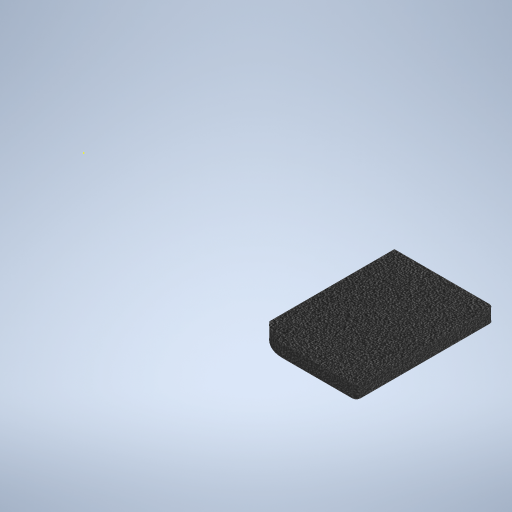
# Autodesk Inventor part: Calco
Saved by Autodesk Inventor 2024 (Build 280153000, 153)
## iProperties
Created: 2024-10-14
Part Number: Calco
Material: Genérico
Document SubType Name: Modeling
Designer: robof
Density: 1 g/cm^3
Appearance: Padrão
Author: robof
Autodesk Inventor part; units mm, degrees
ref_plane "YZ Plane" through (0, 0, 0) normal (1, 0, 0) x (0, 1, 0)
ref_plane "XZ Plane" through (0, 0, 0) normal (0, 1, 0) x (-1, 0, 0)
ref_plane "XY Plane" through (0, 0, 0) normal (0, 0, 1) x (1, 0, 0)
sketch "Esboço1" plane through (0, 0, 0) normal (0, 1, 0) x (-1, 0, 0)
  line L0 (0, 0) -> (-160, 0)
  line L1 (-160, 0) -> (-160, -34)
  line L2 (-160, -34) -> (0, -34)
  line L3 (0, -34) -> (0, 0)
  line L4 (0, 0) -> (-4, 0)
  line L5 (-4, 0) -> (-62.5, 0)
  line L6 (-160, -34) -> (-160, 31)
  line L7 (-160, -34) -> (-117, -34)
  line L8 (-117, -34) -> (-117, 31)
  line L9 (-117, 31) -> (-160, 31)
  line L10 (-160, 31) -> (-160, -34)
  arc A0 (-117, 31) -> (-62.5, 0) centre (-62.5, 63.4073) ccw
  dimension "d0" = 160
  dimension "d1" = 34
  dimension "d2" = 4
  dimension "d3" = 58.5
  dimension "d4" = 65
  dimension "d5" = 43
  constraints: 22 end point, 4 parallel, 3 point on line, 2 horizontal, 2 perpendicular, 2 point on circle, 1 centre point, 1 tangent
  measures "d0" distance of L2.end L1.end
  measures "d1" distance of L1.end L0.end
  measures "d2" distance of L0.start L4.end
  measures "d3" distance of L4.end L5.end
  measures "d4" distance of L1.end L6.end
  measures "d5" distance of L9.end L8.end
extrude "Extrusão1" add sketch "Esboço1" along normal blind 1
fillet "Arredondamento1" radius 2 4 edges at (160, 0.5, 31) (160, 0.5, -34) (0, 0.5, 0) (0, 0.5, -34)
fillet "Arredondamento2" radius 15 1 edges at (117, 0.5, 31)
sketch "Esboço5" plane through (0, 1, 0) normal (0, 1, 0) x (1, 0, 0)
  line L0 (160, -29) -> (160, 32) projected
  line L1 (160, -21.1735) -> (160, -7.1735)
  line L2 (160, -21.1735) -> (146, -21.1735)
  line L3 (124.952, -31) -> (158, -31) projected
  line L4 (146, -31) -> (139, -31)
  line L5 (146, -31) -> (146, -24)
  circle A0 centre (146, -24) radius 3.5
  line L6 (146, -24) -> (130, -24)
  circle A1 centre (130, -24) radius 3.5
  line L7 (146, -24) -> (146, 8)
  circle A2 centre (146, 8) radius 3.5
  line L8 (146, 8) -> (130, 8)
  circle A3 centre (130, 8) radius 3.5
  point P0 (0, 0)
  dimension "d32" = 14
  dimension "d33" = 14
  dimension "d34" = 7
  dimension "d35" = 7
  dimension "d36" = 7
  dimension "d37" = 16
  dimension "d38" = 7
  dimension "d39" = 32
  dimension "d40" = 7
  dimension "d41" = 7
  constraints: 14 end point, 4 centre point, 4 coincident, 4 point on line, 3 horizontal, 2 vertical
  measures "d32" distance of L1.start L1.end
  measures "d33" distance of L1.start L2.end
  measures "d34" distance of L4.start L4.end
  measures "d35" distance of L4.start L5.end
  measures "d36" diameter of A0
  measures "d37" distance of L6.start L6.end
  measures "d38" diameter of A1
  measures "d39" distance of L6.start L7.end
  measures "d40" diameter of A2
  measures "d41" diameter of A3
extrude "Extrusão3" add sketch "Esboço5" along normal blind 1
sketch "Esboço6" plane through (130, 2, -8) normal (0, 1, 0) x (1, 0, 0)
  circle A0 centre (0, 0) radius 2.25
  circle A1 centre (16, 0) radius 3.5 projected
  circle A2 centre (16, 0) radius 2.25
  circle A3 centre (0, -32) radius 3.5 projected
  circle A4 centre (0, -32) radius 2.25
  circle A5 centre (16, -32) radius 3.5 projected
  circle A6 centre (16, -32) radius 2.25
  point P0 (-130, -8)
  dimension "d44" = 4.5
  dimension "d45" = 4.5
  dimension "d46" = 4.5
  dimension "d47" = 4.5
  constraints: 4 centre point, 3 coincident
  measures "d44" diameter of A0
  measures "d45" diameter of A2
  measures "d46" diameter of A4
  measures "d47" diameter of A6
extrude "Extrusão4" add sketch "Esboço6" along normal blind 2.5 contours A0 | A2 | A4 | A6
sketch "Esboço7" plane through (130, 4.5, -8) normal (0, 1, 0) x (1, 0, 0)
  circle A0 centre (0, 0) radius 2.25 projected
  line L0 (-0.7066, -1.2286) -> (-1.4173, -0.0023)
  line L1 (-1.4173, -0.0023) -> (-0.7107, 1.2262)
  line L2 (-0.7107, 1.2262) -> (0.7066, 1.2286)
  line L3 (0.7066, 1.2286) -> (1.4173, 0.0023)
  line L4 (1.4173, 0.0023) -> (0.7107, -1.2262)
  line L5 (0.7107, -1.2262) -> (-0.7066, -1.2286)
  line L6 (0, 0) -> (8, 0)
  line L7 (8, 0) -> (8, -3.5397)
  circle A1 centre (16, 0) radius 2.25
  line L8 (16.7066, -1.2286) -> (17.4173, -0.0023)
  line L9 (17.4173, -0.0023) -> (16.7107, 1.2262)
  line L10 (16.7107, 1.2262) -> (15.2934, 1.2286)
  line L11 (15.2934, 1.2286) -> (14.5827, 0.0023)
  line L12 (14.5827, 0.0023) -> (15.2893, -1.2262)
  line L13 (15.2893, -1.2262) -> (16.7066, -1.2286)
  line L14 (0, 0) -> (0, -16)
  line L15 (0, -16) -> (6.7888, -16)
  circle A2 centre (0, -32) radius 2.25
  line L16 (-0.7066, -30.7714) -> (-1.4173, -31.9977)
  line L17 (-1.4173, -31.9977) -> (-0.7107, -33.2262)
  line L18 (-0.7107, -33.2262) -> (0.7066, -33.2286)
  line L19 (0.7066, -33.2286) -> (1.4173, -32.0023)
  line L20 (1.4173, -32.0023) -> (0.7107, -30.7738)
  line L21 (0.7107, -30.7738) -> (-0.7066, -30.7714)
  circle A3 centre (16, -32) radius 2.25
  line L22 (16.7066, -30.7714) -> (17.4173, -31.9977)
  line L23 (17.4173, -31.9977) -> (16.7107, -33.2262)
  line L24 (16.7107, -33.2262) -> (15.2934, -33.2286)
  line L25 (15.2934, -33.2286) -> (14.5827, -32.0023)
  line L26 (14.5827, -32.0023) -> (15.2893, -30.7738)
  line L27 (15.2893, -30.7738) -> (16.7066, -30.7714)
  point P0 (-130, -8)
  dimension "d50" = 8
  dimension "d51" = 16
  constraints: 56 end point, 24 symmetric about line, 4 coincident, 3 centre point, 2 perpendicular, 1 horizontal, 1 vertical, 16 other
  measures "d50" distance of L6.start L6.end
  measures "d51" distance of L6.start L14.end
extrude "Extrusão5" cut sketch "Esboço7" against normal blind 1.5 contours L6 L14 L5 L0 L1 L2 L3 L4 | L4 L5 L14 L6 | L13 L12 L11 L10 L9 L8 | L21 L20 L19 L18 L17 L16 | L22 L23 L24 L25 L26 L27
sketch "Esboço8" plane through (0, 1, 0) normal (0, 1, 0) x (1, 0, 0)
  line L0 (0, 0) -> (6, 0)
  line L1 (2, 0) -> (62.5, 0) projected
  line L2 (6, 0) -> (-1.5, 0)
  line L3 (6, 0) -> (6, 7.5)
  circle A0 centre (6, 7.5) radius 2.25
  line L4 (0, 32) -> (0, 2) projected
  line L5 (0, 17) -> (13.7618, 17)
  circle A1 centre (6, 26.5) radius 2.25
  dimension "d54" = 6
  dimension "d55" = 7.5
  dimension "d56" = 7.5
  dimension "d57" = 4.5
  constraints: 8 end point, 2 centre point, 2 point on line, 1 coincident, 1 horizontal, 1 midpoint, 1 symmetric about line, 1 vertical, 1 other
  measures "d54" distance of L0.start L0.end
  measures "d55" distance of L0.end L2.end
  measures "d56" distance of L0.end L3.end
  measures "d57" diameter of A0
extrude "Extrusão6" cut sketch "Esboço8" against normal blind 0.1
sketch "Esboço9" plane through (6, 0.9, -26.5) normal (0, 1, 0) x (1, 0, 0)
  circle A0 centre (0, -19) radius 2.25 projected
  line L0 (0, -19) -> (0.25, -19)
  line L1 (0.25, -19) -> (0.25, -20.5)
  line L2 (0.25, -20.5) -> (0, -20.5)
  line L3 (0, -20.5) -> (0, -19)
  line L4 (0, -20.5) -> (-0.25, -20.5)
  line L5 (-0.25, -20.5) -> (-0.25, -19)
  line L6 (-0.25, -19) -> (0, -19)
  line L7 (0, -19) -> (0, -20.5)
  line L8 (0.25, -20.5) -> (-0.25, -20.5)
  line L9 (-0.25, -20.5) -> (-0.25, -17.5)
  line L10 (-0.25, -17.5) -> (0.25, -17.5)
  line L11 (0.25, -17.5) -> (0.25, -20.5)
  line L12 (0, -19) -> (1.5, -19)
  line L13 (1.5, -19) -> (1.5, -18.75)
  line L14 (1.5, -18.75) -> (0, -18.75)
  line L15 (0, -18.75) -> (0, -19)
  line L16 (1.5, -18.75) -> (-1.5, -18.75)
  line L17 (-1.5, -18.75) -> (-1.5, -19.25)
  line L18 (-1.5, -19.25) -> (1.5, -19.25)
  line L19 (1.5, -19.25) -> (1.5, -18.75)
  line L20 (-6, 5.5) -> (-6, -24.5) projected
  line L21 (-6, -9.5) -> (4.7143, -9.5)
  line L22 (0, 0) -> (0.25, 0)
  line L23 (0.25, 0) -> (0.25, 1.5)
  line L24 (0.25, 1.5) -> (0, 1.5)
  line L25 (0, 1.5) -> (0, 0)
  line L26 (0, 1.5) -> (-0.25, 1.5)
  line L27 (-0.25, 1.5) -> (-0.25, 0)
  line L28 (-0.25, 0) -> (0, 0)
  line L29 (0, 0) -> (0, 1.5)
  line L30 (0.25, 1.5) -> (-0.25, 1.5)
  line L31 (-0.25, 1.5) -> (-0.25, -1.5)
  line L32 (-0.25, -1.5) -> (0.25, -1.5)
  line L33 (0.25, -1.5) -> (0.25, 1.5)
  line L34 (0, 0) -> (1.5, 0)
  line L35 (1.5, 0) -> (1.5, -0.25)
  line L36 (1.5, -0.25) -> (0, -0.25)
  line L37 (0, -0.25) -> (0, 0)
  line L38 (1.5, -0.25) -> (-1.5, -0.25)
  line L39 (-1.5, -0.25) -> (-1.5, 0.25)
  line L40 (-1.5, 0.25) -> (1.5, 0.25)
  line L41 (1.5, 0.25) -> (1.5, -0.25)
  point P0 (-6, -26.5)
  point P1 (-0.25, -19.25)
  point P2 (0.25, -19.25)
  point P3 (0.25, -18.75)
  point P4 (-0.25, -18.75)
  point P5 (0.25, 0.25)
  point P6 (-0.25, 0.25)
  point P7 (-0.25, -0.25)
  point P8 (0.25, -0.25)
  dimension "d60" = 0.25
  dimension "d61" = 1.5
  dimension "d62" = 0.25
  dimension "d63" = 3
  dimension "d64" = 1.5
  dimension "d65" = 0.25
  dimension "d66" = 3
  dimension "d67" = 0.5
  constraints: 82 end point, 16 symmetric about line, 10 parallel, 6 horizontal, 5 perpendicular, 4 point on line, 1 midpoint
  measures "d60" distance of L1.end L2.end
  measures "d61" distance of L0.end L1.end
  measures "d62" distance of L5.end L6.end
  measures "d63" distance of L8.end L9.end
  measures "d64" distance of L14.end L13.end
  measures "d65" distance of L13.end L12.end
  measures "d66" distance of L18.end L17.end
  measures "d67" distance of L17.end L16.end
extrude "Extrusão7" cut sketch "Esboço9" against normal blind 0.1 contours L15 L14 L11 L0 | L0 L1 L18 L3 | L3 L18 L5 L6 | L6 L9 L16 L15 | L12 L19 L18 L1 | L11 L14 L13 L12 | L18 L1 L2 L3 | L3 L4 L5 L18 | L5 L18 L17 L16 L9 | L16 L9 L10 L11 L14 | L25 L40 L23 L22 | L28 L27 L40 L25 | L37 L38 L31 L28 | L22 L33 L36 L37 | L34 L35 L36 L33 | L23 L40 L41 L34 | L40 L27 L26 L25 | L25 L24 L23 L40 | L31 L38 L39 L40 L27 | L36 L33 L32 L31 L38
sketch "Esboço10" plane through (6, 0.9, -26.5) normal (0, 1, 0) x (1, 0, 0)
  line L0 (0, 0) -> (52, 0)
  circle A0 centre (52, 0) radius 2.25
  circle A1 centre (0, -19) radius 2.25 projected
  line L1 (0, -19) -> (52, -19)
  circle A2 centre (52, -19) radius 2.25
  point P0 (-6, -26.5)
  dimension "d70" = 52
  dimension "d71" = 4.5
  dimension "d72" = 52
  dimension "d73" = 4.5
  constraints: 4 end point, 2 centre point, 2 coincident, 1 horizontal, 1 parallel
  measures "d70" distance of L0.start L0.end
  measures "d71" diameter of A0
  measures "d72" distance of L1.start L1.end
  measures "d73" diameter of A2
extrude "Extrusão8" cut sketch "Esboço10" along normal blind 2 contours A0 | A2
sketch "Esboço11" plane through (58, 0.9, -26.5) normal (0, 1, 0) x (1, 0, 0)
  line L0 (0, 0) -> (0.25, 0)
  line L1 (0.25, 0) -> (0.25, 1.5)
  line L2 (0.25, 1.5) -> (0, 1.5)
  line L3 (0, 1.5) -> (0, 0)
  line L4 (0.25, 1.5) -> (-0.25, 1.5)
  line L5 (-0.25, 1.5) -> (-0.25, -1.5)
  line L6 (-0.25, -1.5) -> (0.25, -1.5)
  line L7 (0.25, -1.5) -> (0.25, 1.5)
  line L8 (0, 0) -> (1.5, 0)
  line L9 (1.5, 0) -> (1.5, 0.25)
  line L10 (1.5, 0.25) -> (0, 0.25)
  line L11 (0, 0.25) -> (0, 0)
  line L12 (1.5, 0.25) -> (-1.5, 0.25)
  line L13 (-1.5, 0.25) -> (-1.5, -0.25)
  line L14 (-1.5, -0.25) -> (1.5, -0.25)
  line L15 (1.5, -0.25) -> (1.5, 0.25)
  line L16 (-58, 5.5) -> (-58, -24.5) projected
  line L17 (-58, -9.5) -> (-46.2393, -9.5)
  line L18 (0, -19) -> (0.25, -19)
  line L19 (0.25, -19) -> (0.25, -20.5)
  line L20 (0.25, -20.5) -> (0, -20.5)
  line L21 (0, -20.5) -> (0, -19)
  line L22 (0.25, -20.5) -> (-0.25, -20.5)
  line L23 (-0.25, -20.5) -> (-0.25, -17.5)
  line L24 (-0.25, -17.5) -> (0.25, -17.5)
  line L25 (0.25, -17.5) -> (0.25, -20.5)
  line L26 (0, -19) -> (1.5, -19)
  line L27 (1.5, -19) -> (1.5, -19.25)
  line L28 (1.5, -19.25) -> (0, -19.25)
  line L29 (0, -19.25) -> (0, -19)
  line L30 (1.5, -19.25) -> (-1.5, -19.25)
  line L31 (-1.5, -19.25) -> (-1.5, -18.75)
  line L32 (-1.5, -18.75) -> (1.5, -18.75)
  line L33 (1.5, -18.75) -> (1.5, -19.25)
  point P0 (-58, -26.5)
  point P1 (0.25, -0.25)
  point P2 (1.5, 0)
  point P3 (0.25, 0.25)
  point P4 (0, 1.5)
  point P5 (-0.25, 0.25)
  point P6 (-0.25, -0.25)
  point P7 (0.25, -19.25)
  point P8 (1.5, -19)
  point P9 (0.25, -18.75)
  point P10 (-0.25, -18.75)
  point P11 (-0.25, -19.25)
  dimension "d76" = 0.25
  dimension "d77" = 1.5
  dimension "d78" = 0.5
  dimension "d79" = 3
  dimension "d80" = 1.5
  dimension "d81" = 0.25
  dimension "d82" = 3
  dimension "d83" = 0.5
  constraints: 66 end point, 13 symmetric about line, 8 parallel, 5 horizontal, 4 perpendicular, 1 midpoint
  measures "d76" distance of L2.end L1.end
  measures "d77" distance of L1.end L0.end
  measures "d78" distance of L6.end L5.end
  measures "d79" distance of L5.end L4.end
  measures "d80" distance of L10.end L9.end
  measures "d81" distance of L9.end L8.end
  measures "d82" distance of L14.end L13.end
  measures "d83" distance of L13.end L12.end
extrude "Extrusão9" cut sketch "Esboço11" against normal blind 0.1
sketch "Esboço12" plane through (0, 0, 0) normal (0, -1, 0) x (1, 0, 0)
  arc A0 (124.952, 31) -> (113.0044, 25.0694) centre (124.952, 16) ccw projected
  line L0 (160, -34) -> (124.952, -34)
  line L1 (124.952, -34) -> (124.952, 31)
  line L2 (124.952, 31) -> (160, 31)
  line L3 (160, 31) -> (160, -34)
  line L4 (113.0044, 25.0694) -> (124.952, 25.0694)
  line L5 (124.952, 25.0694) -> (124.952, -34)
  line L6 (124.952, -34) -> (113.0044, -34)
  line L7 (113.0044, -34) -> (113.0044, 25.0694)
  arc A1 (124.952, 31) -> (113.0044, 25.0694) centre (124.952, 16) ccw
  point P0 (0, 0)
  constraints: 16 end point, 4 parallel, 2 horizontal, 2 perpendicular, 2 point on circle, 1 centre point
extrude "Extrusão10" add sketch "Esboço12" along normal blind 5
sketch "Esboço13" plane through (0, 1, 0) normal (0, 1, 0) x (1, 0, 0)
  point P0 (0, 0)
sketch "Esboço14" plane through (0, -5, 0) normal (0, -1, 0) x (1, 0, 0)
  arc A0 (160, 29) -> (158, 31) centre (158, 29) ccw projected
  circle A1 centre (158, 29) radius 2
  arc A2 (158, -34) -> (160, -32) centre (158, -32) ccw projected
  circle A3 centre (158, -32) radius 2
  line L0 (160, 31) -> (124.952, 31) projected
  line L1 (158, 29) -> (160, 29)
  line L2 (160, 29) -> (160, 31)
  line L3 (160, 31) -> (158, 31)
  line L4 (158, 31) -> (158, 29)
  line L5 (158, -32) -> (160, -32)
  line L6 (160, -32) -> (160, -34)
  line L7 (160, -34) -> (158, -34)
  line L8 (158, -34) -> (158, -32)
  point P0 (0, 0)
  constraints: 16 end point, 4 parallel, 2 centre point, 2 coincident, 2 horizontal, 2 perpendicular, 1 point on line
extrude "Extrusão11" cut sketch "Esboço14" against normal blind 20 contours A0 L0 L2 | A2 L6 L7
sketch "Esboço15" plane through (158, 1, -34) normal (0, 0, -1) x (-1, 0, 0)
  line L0 (44.9956, -1) -> (95.5, -1) projected
  line L1 (44.9956, -1) -> (158, -1)
  line L2 (158, -1) -> (158, 2.7863)
  line L3 (158, 2.7863) -> (44.9956, 2.7863)
  line L4 (44.9956, 2.7863) -> (44.9956, -1)
  line L5 (-2, 0) -> (0, 0) projected
  line L6 (-2, 0) -> (44.9956, 0)
  line L7 (44.9956, 0) -> (44.9956, 5.0916)
  line L8 (44.9956, 5.0916) -> (-2, 5.0916)
  line L9 (-2, 5.0916) -> (-2, 0)
  point P0 (44.9956, 0)
  constraints: 16 end point, 4 parallel, 2 horizontal, 2 perpendicular, 1 point on line
extrude "Extrusão12" cut sketch "Esboço15" against normal blind 66
